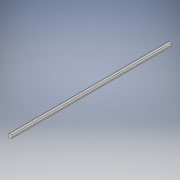
# Autodesk Inventor part: hex shaft 1
Saved by Autodesk Inventor 2018 (Build 220112000, 112)
## iProperties
Created: 2020-01-22
Part Number: hex shaft 1
Material: Generic
Document SubType Name: Modeling
Designer: s-2513225
Density: 1 g/cm^3
Appearance: Default
Author: s-2513225
Autodesk Inventor part; units mm, degrees
ref_plane "YZ Plane" through (0, 0, 0) normal (1, 0, 0) x (0, 1, 0)
ref_plane "XZ Plane" through (0, 0, 0) normal (0, 1, 0) x (-1, 0, 0)
ref_plane "XY Plane" through (0, 0, 0) normal (0, 0, 1) x (1, 0, 0)
sketch "Sketch1" plane through (0, 0, 0) normal (0, 0, 1) x (1, 0, 0)
  line L0 (1.0025, -6.7997) -> (-4.0992, -5.517)
  line L1 (-4.0992, -5.517) -> (-6.7997, -1.0025)
  line L2 (-6.7997, -1.0025) -> (-5.517, 4.0992)
  line L3 (-5.517, 4.0992) -> (-1.0025, 6.7997)
  line L4 (-1.0025, 6.7997) -> (4.0992, 5.517)
  line L5 (4.0992, 5.517) -> (6.7997, 1.0025)
  line L6 (6.7997, 1.0025) -> (5.517, -4.0992)
  line L7 (5.517, -4.0992) -> (1.0025, -6.7997)
  point P0 (0, 0)
  point P1 (0, 0)
  dimension "d0" = 12.7
  constraints: 16 end point, 1 coincident, 17 other
  measures "d0" distance between parallel lines of L0 L4
extrude "Extrusion1" add sketch "Sketch1" along normal blind 533.4
body "Solid1"
